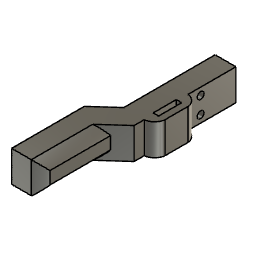
mors_gauche (Autodesk Fusion 360 design; units mm, degrees)
Autodesk Fusion 360 part; units mm, degrees
sketch "Esquisse2" plane through (0, 0, 0) normal (0, 0, 1) x (1, 0, 0)
  line L0 (0, 0) -> (10, 0)
  line L1 (10, 0) -> (10, 30)
  line L2 (0, 0) -> (0, 35)
  line L3 (20, 39) -> (20, 88)
  line L4 (20, 88) -> (10, 88)
  line L5 (10, 88) -> (10, 44)
  line L6 (0, 35) -> (10, 44)
  line L7 (10, 30) -> (20, 39)
  dimension "d1" = 10
  dimension "d2" = 30
  dimension "d3" = 35
  dimension "d5" = 49
  dimension "d6" = 10
  dimension "d8" = 10
  dimension "d9" = 14
  constraint coincident L0.start L2.start
  constraint horizontal L0
  constraint perpendicular L0 L1
  constraint perpendicular L0 L2
  constraint perpendicular L3 L4
  constraint perpendicular L4 L5
  constraint parallel L6 L7
  measures "d1" distance of L0.start L0.end
  measures "d2" distance of L0.end L1.end
  measures "d3" distance of L0.start L2.end
  measures "d5" distance of L3.start L3.end
  measures "d6" distance of L3.end L4.end
  measures "d8" horizontal distance of L1.end L3.start
  measures "d9" distance of L1.end L5.end
extrude "Extrusion1" add sketch "Esquisse2" along normal blind 15
move_face "DécalerLesFaces1" offset 4 1 faces at (10, 10, 10)
fillet "Congé1" radius 4.5 tangency weight 0.1 3 edges at (14, 16.8, 15) (14, 0, 7.5) (14, 16.8, 0)
sketch "Esquisse3" plane through (20, 0, 0) normal (1, 0, 0) x (0, 1, 0)
  line L0 (39, 0) -> (88, 0)
  line L1 (88, 0) -> (88, 15)
  line L2 (88, 15) -> (39, 15)
  line L3 (39, 15) -> (39, 0)
  circle A0 centre (71, 3.5) radius 1.65
  circle A1 centre (71, 11.5) radius 1.65
  line L4 (69.4856, 15) -> (69.4856, 0)
  line L5 (43.9058, 15) -> (64.9058, 15)
  line L6 (64.9058, 15) -> (64.9058, 0)
  line L7 (64.9058, 0) -> (43.9058, 0)
  line L8 (43.9058, 0) -> (43.9058, 15)
  dimension "d17" = 3.3
  dimension "d19" = 3.3
  dimension "d20" = 17
  dimension "d21" = 17
  dimension "d37" = 21
  constraint coincident L2 L4.start
  constraint coincident L0 L4.end
  constraint perpendicular L0 L4
  constraint horizontal L5
  constraint vertical L6
  constraint horizontal L7
  constraint vertical L8
  constraint coincident L0 L6.end
  constraint coincident L2 L5.start
  measures "d17" diameter of A0
  measures "d19" diameter of A1
  measures "d20" distance of L1 A0.centre
  measures "d21" distance of L1 A1.centre
  measures "d37" distance of L6 L8
extrude "Extrusion4" add sketch "Esquisse3" along normal blind 6 contours L0 L2 L5 L6 L7 L8
sketch "Esquisse7" plane through (0, 0, 0) normal (0, 0, -1) x (1, 0, 0)
  line L0 (20, -39) -> (9.5, -29.55)
  line L1 (9.5, 0) -> (9.5, -29.55)
  line L2 (9.5, 0) -> (0, 0)
  line L3 (0, 0) -> (0, -35)
  line L4 (0, -35) -> (10, -44)
  line L5 (10, -44) -> (10, -88)
  line L6 (10, -88) -> (20, -88)
  line L7 (20, -88) -> (20, -64.9058)
  line L8 (20, -64.9058) -> (26, -64.9058)
  line L9 (26, -64.9058) -> (26, -43.9058)
  line L10 (26, -43.9058) -> (20, -43.9058)
  line L11 (20, -43.9058) -> (20, -39)
  line L12 (21.9204, -48.8558) -> (19.3204, -48.8558)
  line L13 (19.3204, -48.8558) -> (19.3204, -59.9558)
  line L14 (19.3204, -59.9558) -> (21.9204, -59.9558)
  line L15 (21.9204, -59.9558) -> (21.9204, -48.8558)
  line L16 (21.9204, -54.4058) -> (19.3204, -54.4058)
  dimension "d43" = 2.6
  dimension "d44" = 11.1
  dimension "d46" = 10.5
  constraint horizontal L12
  constraint vertical L13
  constraint horizontal L14
  constraint vertical L15
  constraint midpoint L15 L16.start
  constraint midpoint L13 L16.end
  measures "d43" distance of L12.start L12.end
  measures "d44" distance of L12.start L14.end
  measures "d46" distance of L8 L16
extrude "Extrusion5" cut sketch "Esquisse7" against normal blind 15 contours L12 L13 L15 L16 | L13 L14 L15 L16
extrude "Extrusion6" cut 1 faces at (26, 50.9058, 10) along direction (-1, 0, 0) blind 1
fillet "Congé3" radius 5 tangency weight 0.77596 2 edges at (25, 64.9058, 7.5) (25, 43.9058, 7.5)
extrude "Extrusion7" cut sketch "Esquisse3" against normal blind 15 contours A0 L4 | A0 L4 | A1 L4 | A1 L4
sketch "Esquisse8" plane through (0, 0, 0) normal (-1, 0, 0) x (0, -1, 0)
  line L0 (-35, 0) -> (0, 0)
  line L1 (0, 0) -> (0, 15)
  line L2 (0, 15) -> (-35, 15)
  line L3 (-35, 15) -> (-35, 0)
  circle A0 centre (-32.5, 2.5) radius 2.5
  circle A1 centre (-27.5, 2.5) radius 2.5
  circle A2 centre (-22.5, 2.5) radius 2.5
  circle A3 centre (-17.5, 2.5) radius 2.5
  circle A4 centre (-12.5, 2.5) radius 2.5
  circle A5 centre (-7.5, 2.5) radius 2.5
  circle A6 centre (-2.5, 2.5) radius 2.5
  circle A7 centre (-32.5, 7.5) radius 2.5
  circle A8 centre (-27.5, 7.5) radius 2.5
  circle A9 centre (-22.5, 7.5) radius 2.5
  circle A10 centre (-17.5, 7.5) radius 2.5
  circle A11 centre (-12.5, 7.5) radius 2.5
  circle A12 centre (-7.5, 7.5) radius 2.5
  circle A13 centre (-2.5, 7.5) radius 2.5
  circle A14 centre (-32.5, 12.5) radius 2.5
  circle A15 centre (-27.5, 12.5) radius 2.5
  circle A16 centre (-22.5, 12.5) radius 2.5
  circle A17 centre (-17.5, 12.5) radius 2.5
  circle A18 centre (-12.5, 12.5) radius 2.5
  circle A19 centre (-7.5, 12.5) radius 2.5
  circle A20 centre (-2.5, 12.5) radius 2.5
  dimension "d59" = 30
  dimension "d60" = 10
extrude "Extrusion8" add sketch "Esquisse8" along normal blind 1 draft -70 contours A14
extrude "Extrusion9" add sketch "Esquisse8" along normal blind 1 draft -70 contours A15
extrude "Extrusion10" add sketch "Esquisse8" along normal blind 1 draft -70 contours A16 | A17
extrude "Extrusion11" add sketch "Esquisse8" along normal blind 1 draft -70 contours A18
extrude "Extrusion12" add sketch "Esquisse8" along normal blind 1 draft -70 contours A19
extrude "Extrusion13" add sketch "Esquisse8" along normal blind 1 draft -70 contours A20
extrude "Extrusion14" add sketch "Esquisse8" along normal blind 1 draft -70 contours A7
extrude "Extrusion24" add sketch "Esquisse8" along normal blind 1 draft -70 contours A8
extrude "Extrusion25" add sketch "Esquisse8" along normal blind 1 draft -70 contours A9
extrude "Extrusion26" add sketch "Esquisse8" along normal blind 1 draft -70 contours A10
extrude "Extrusion27" add sketch "Esquisse8" along normal blind 1 draft -70 contours A11
extrude "Extrusion28" add sketch "Esquisse8" along normal blind 1 draft -70 contours A12
extrude "Extrusion29" add sketch "Esquisse8" along normal blind 1 draft -70 contours A13
extrude "Extrusion30" add sketch "Esquisse8" along normal blind 1 draft -70 contours A0
extrude "Extrusion31" add sketch "Esquisse8" along normal blind 1 draft -70 contours A1
extrude "Extrusion32" add sketch "Esquisse8" along normal blind 1 draft -70 contours A2
extrude "Extrusion33" add sketch "Esquisse8" along normal blind 1 draft -70 contours A3
extrude "Extrusion34" add sketch "Esquisse8" along normal blind 1 draft -70 contours A4
extrude "Extrusion35" add sketch "Esquisse8" along normal blind 1 draft -70 contours A5
extrude "Extrusion36" add sketch "Esquisse8" along normal blind 1 draft -70 contours A6
extrude "Extrusion15" [suppressed]
extrude "Extrusion16" [suppressed]
extrude "Extrusion17" [suppressed]
extrude "Extrusion18" [suppressed]
extrude "Extrusion19" [suppressed]
extrude "Extrusion20" [suppressed]
extrude "Extrusion21" [suppressed]
extrude "Extrusion22" [suppressed]
extrude "Extrusion23" [suppressed]
extrude "Extrusion3" [suppressed]
extrude "Extrusion2" [suppressed]
fillet "Congé2" [suppressed]
equation "d19 = d17"
equation "d20 = d21"
